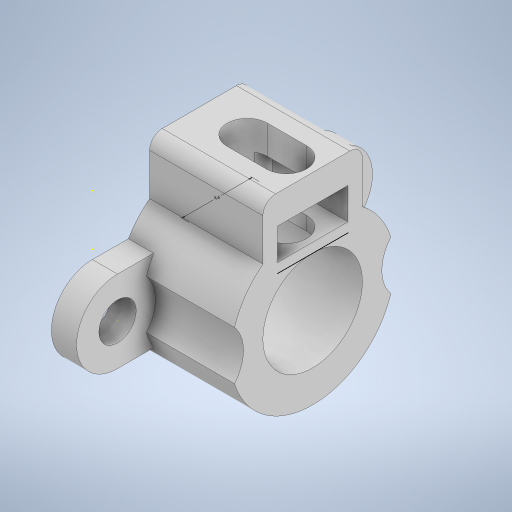
# Autodesk Inventor part: acople2
Saved by Autodesk Inventor 2024 (Build 280153000, 153)
## iProperties
Created: 2024-08-16
Part Number: acople2
Material: Generic
Document SubType Name: Modeling
Designer: David Ricaurte
Density: 1 g/cm^3
Appearance: Default
Author: David Ricaurte
Autodesk Inventor part; units mm, degrees
ref_plane "YZ Plane" through (0, 0, 0) normal (1, 0, 0) x (0, 1, 0)
ref_plane "XZ Plane" through (0, 0, 0) normal (0, 1, 0) x (-1, 0, 0)
ref_plane "XY Plane" through (0, 0, 0) normal (0, 0, 1) x (1, 0, 0)
sketch "Sketch1" plane through (0, 0, 0) normal (1, 0, 0) x (0, 1, 0)
  line L0 (0, 0) -> (0, -17)
  circle A0 centre (0, 0) radius 1.6
  circle A1 centre (0, -17) radius 1.6
  circle A2 centre (0, 0) radius 3.25
  circle A3 centre (0, -17) radius 3.25
  circle A4 centre (0, -8.5) radius 6.5
  line L1 (3.25, 0) -> (3.25, -17)
  line L2 (-3.25, 0) -> (-3.25, -17)
  point P0 (3.25, -14.1292)
  point P1 (3.25, -2.8708)
  point P2 (-3.25, -2.8708)
  point P3 (-3.25, -14.1292)
  dimension "d3" = 6.5
  dimension "d4" = 6.5
  dimension "d0" = 17
  dimension "d1" = 3.2
  dimension "d2" = 3.2
  dimension "d5" = 13
  constraints: 6 end point, 4 coincident, 3 centre point, 2 symmetric about line, 2 vertical, 1 midpoint, 6 other
  measures "d0" distance of L0.start L0.end
  measures "d1" diameter of A0
  measures "d2" diameter of A1
  measures "d5" diameter of A4
extrude "Extrusion1" add sketch "Sketch1" along normal blind 2
sketch "Sketch2" plane through (2, 0, 0) normal (1, 0, 0) x (0, 0, -1)
  arc A0 (14.1292, 3.25) -> (2.8708, 3.25) centre (8.5, 0) ccw projected
  circle A1 centre (8.5, 0) radius 6.5
  circle A2 centre (8.5, 0) radius 3.95
  point P0 (0, 0)
  point P1 (2.8708, 3.25)
  point P2 (14.1292, 3.25)
  dimension "d8" = 7.9
  constraints: 2 centre point, 2 coincident
  measures "d8" diameter of A2
extrude "Extrusion2" add sketch "Sketch2" along normal blind 7
sketch "Sketch3" plane through (2, 0, 0) normal (1, 0, 0) x (0, 0, -1)
  circle A0 centre (0, 0) radius 3
  circle A1 centre (17, 0) radius 1.6 projected
  circle A2 centre (17, 0) radius 3
  dimension "d11" = 6
  dimension "d12" = 6
  constraints: 2 centre point, 2 coincident
  measures "d11" diameter of A0
  measures "d12" diameter of A2
extrude "Extrusion3" cut sketch "Sketch3" along normal through all contours A0 | A1 | A2
sketch "Sketch4" plane through (0, 0, 0) normal (-1, 0, 0) x (0, 0, 1)
  circle A0 centre (-8.5, 0) radius 3.95 projected
  line L0 (-8.5, 0) -> (-8.5, 3.95)
  line L1 (-5.7, 6.45) -> (-11.3, 6.45)
  line L2 (-11.3, 6.45) -> (-11.3, 1.45)
  line L3 (-11.3, 1.45) -> (-5.7, 1.45)
  line L4 (-5.7, 1.45) -> (-5.7, 6.45)
  line L5 (-5.7, 6.45) -> (-11.3, 1.45) construction
  line L6 (-11.3, 6.45) -> (-5.7, 1.45) construction
  line L7 (-11.3, 3.95) -> (-5.7, 3.95)
  line L8 (-12.45, -7.9907) -> (-4.55, -7.9907)
  line L9 (-4.55, -7.9907) -> (-4.55, 7.9907)
  line L10 (-4.55, 7.9907) -> (-12.45, 7.9907)
  line L11 (-12.45, 7.9907) -> (-12.45, -7.9907)
  line L12 (-12.45, -7.9907) -> (-4.55, 7.9907) construction
  line L13 (-4.55, -7.9907) -> (-12.45, 7.9907) construction
  arc A1 (-2.2941, 1.9331) -> (-14.7059, 1.9331) centre (-8.5, 0) ccw projected
  line L14 (-4.55, 5.1621) -> (-12.45, 5.1621)
  point P0 (0, 0)
  point P1 (-5.7, 5.1621)
  point P2 (-5.7, 2.7861)
  point P3 (-4.55, 0)
  dimension "d15" = 5.6
  dimension "d16" = 5
  constraints: 30 end point, 6 midpoint, 4 parallel, 2 horizontal, 2 perpendicular, 2 point on circle, 2 point on line, 1 vertical, 2 other
  measures "d15" distance of L3.end L2.end
  measures "d16" distance of L2.end L1.end
extrude "Extrusion4" add sketch "Sketch4" against normal blind 9 contours A0 L4 L14 L9 | A1 L4 L1 L2 L11 L10 L9 | L14 L4 A1 | A1 L2 L14 | A1 L1 L4 | L4 L14 L2 A1 L1 | L2 L1 A1 | L1 A1
sketch "Sketch5" plane through (9, 0, 0) normal (1, 0, 0) x (0, 0, -1)
  circle A0 centre (8.5, 0) radius 3.95 projected
  line L0 (8.5, 0) -> (8.5, 3.95)
  line L1 (5.7, 1.45) -> (11.3, 1.45)
  line L2 (11.3, 1.45) -> (11.3, 6.45)
  line L3 (11.3, 6.45) -> (5.7, 6.45)
  line L4 (5.7, 6.45) -> (5.7, 1.45)
  line L5 (5.7, 1.45) -> (11.3, 6.45) construction
  line L6 (11.3, 1.45) -> (5.7, 6.45) construction
  line L7 (8.5, 3.95) -> (5.7, 3.95)
  line L8 (5.7, 3.95) -> (11.3, 3.95)
  point P0 (0, 0)
  dimension "d19" = 5.6
  dimension "d20" = 5
  constraints: 18 end point, 4 midpoint, 2 parallel, 1 horizontal, 1 perpendicular, 1 vertical, 1 vertical alignment, 1 other
  measures "d19" distance of L3.end L2.end
  measures "d20" distance of L2.end L1.end
extrude "Extrusion5" cut sketch "Sketch5" against normal blind 6 contours L7 L4 L3 L2 L8
sketch "Sketch6" plane through (0, 7.9907, -4.55) normal (0, 1, 0) x (1, 0, 0)
  point P0 (0, -4.55)
sketch "Sketch7" plane through (0, 7.9907, -4.55) normal (0, 1, 0) x (1, 0, 0)
  line L0 (9, 3.95) -> (3, 3.95) projected
  line L1 (3.8147, 3.95) -> (6.916, 3.95) construction
  line L2 (3.8147, 2.35) -> (6.916, 2.35)
  line L3 (6.916, 5.55) -> (3.8147, 5.55)
  arc A0 (3.8147, 5.55) -> (3.8147, 2.35) centre (3.8147, 3.95) ccw
  arc A1 (6.916, 2.35) -> (6.916, 5.55) centre (6.916, 3.95) ccw
  point P0 (0, -4.55)
  point P1 (5.3654, 3.95)
  dimension "d23" = 3.2
  constraints: 8 end point, 4 point on circle, 4 tangent, 2 centre point, 1 midpoint, 1 parallel
  measures "d23" diameter of A1
sketch "Sketch8" plane through (9, 3.95, -8.5) normal (0, 1, 0) x (1, 0, 0)
  line L0 (0, 0) -> (0, -2.8) projected
  line L1 (-7, -3.95) -> (-7, 3.95) projected
  line L2 (0, -2.8) -> (-7, -2.8)
  line L3 (-7, -2.8) -> (-7, 2.7358)
  line L4 (0, -2.8) -> (-7, -2.8)
  line L5 (-7, -2.8) -> (-7, 2.8)
  line L6 (-7, 2.8) -> (0, 2.8)
  line L7 (0, 2.8) -> (0, -2.8)
  point P0 (-9, -8.5)
  dimension "d28" = 5.6
  constraints: 12 end point, 2 horizontal, 2 parallel, 2 perpendicular, 2 point on line
  measures "d28" distance of L4.end L5.end
sketch "Sketch9" plane through (9, 0, 0) normal (1, 0, 0) x (0, 0, -1)
  line L0 (5.7, 3.95) -> (5.7, 6.45) projected
  line L1 (5.7, 6.45) -> (11.3, 6.45)
  line L2 (11.3, 6.45) -> (11.3, 7.2)
  line L3 (11.3, 7.2) -> (5.7, 7.2)
  line L4 (5.7, 7.2) -> (5.7, 6.45)
  point P0 (0, 0)
  dimension "d29" = 0.75
  constraints: 8 end point, 2 parallel, 1 horizontal, 1 perpendicular
  measures "d29" distance of L2.end L1.end
extrude "Extrusion8" cut sketch "Sketch9" against normal blind 6
sketch "Sketch10" plane through (9, 0, 0) normal (1, 0, 0) x (0, 0, -1)
  line L0 (11.3, 7.2) -> (11.3, 3.95) projected
  line L1 (5.7, 3.95) -> (5.7, 7.2) projected
  line L2 (11.3, 3.95) -> (5.7, 3.95)
  line L3 (5.7, 3.95) -> (5.7, 4.7)
  line L4 (5.7, 4.7) -> (11.3, 4.7)
  line L5 (11.3, 4.7) -> (11.3, 3.95)
  point P0 (0, 0)
  dimension "d32" = 0.75
  constraints: 8 end point, 2 parallel, 1 horizontal, 1 perpendicular, 1 point on line
  measures "d32" distance of L2.end L3.end
extrude "Extrusion9" add sketch "Sketch10" against normal blind 6
sketch "Sketch11" plane through (0, 7.9907, -4.55) normal (0, 1, 0) x (1, 0, 0)
  line L0 (0, -1.6792) -> (0, 0) projected
  line L1 (9, 7.9) -> (9, 10.1559) projected
  line L2 (0, 0) -> (9, 0)
  line L3 (9, 0) -> (9, 7.9)
  line L4 (9, 7.9) -> (0, 7.9)
  line L5 (0, 7.9) -> (0, 0)
  point P0 (0, -4.55)
  constraints: 8 end point, 2 parallel, 1 horizontal, 1 perpendicular
extrude "Extrusion11" add sketch "Sketch11" along normal blind 1.5
extrude "Extrusion12" cut sketch "Sketch7" along normal mid plane 10
fillet "Fillet1" radius 1 2 edges at (4.5, 9.4907, -4.55) (4.5, 9.4907, -12.45)
sketch "Sketch12" plane through (2, 0, 0) normal (1, 0, 0) x (0, 0, -1)
  circle A0 centre (0, 0) radius 1.6 projected
  circle A1 centre (0, 0) radius 2.1992
  circle A2 centre (17, 0) radius 1.6 projected
  circle A3 centre (17, 0) radius 2.2664
  constraints: 2 centre point, 2 coincident
extrude "Extrusion13" add sketch "Sketch12" against normal blind 2 contours A0 | A1 | A2 | A3
sketch "Sketch13" plane through (2, 0, 0) normal (1, 0, 0) x (0, 0, -1)
  circle A0 centre (0, 0) radius 1.475
  arc A1 (17, -3.25) -> (17, 3.25) centre (17, 0) ccw projected
  circle A2 centre (17, 0) radius 1.475
  dimension "d44" = 2.95
  dimension "d45" = 2.95
  constraints: 2 centre point, 2 coincident
  measures "d44" diameter of A0
  measures "d45" diameter of A2
extrude "Extrusion14" cut sketch "Sketch13" against normal blind 2
sketch "Sketch14" plane through (2, 0, -8.5) normal (1, 0, 0) x (0, 0, -1)
  circle A0 centre (0, 0) radius 3.95
  point P0 (-8.5, 0)
  constraints: 1 centre point
extrude "Extrusion15" cut sketch "Sketch14" against normal blind 10
sketch "Sketch15" plane through (2, 0, 0) normal (1, 0, 0) x (0, 0, -1)
  point P0 (0, 0)
body "Solid1"
